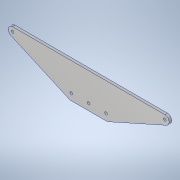
# Autodesk Inventor part: ハンド_上側板
Saved by Autodesk Inventor 2021 (Build 250183000, 183)
## iProperties
Created: 2021-12-06
Part Number: ハンド_上側板
Material: アルミニウム 6061
Document SubType Name: Modeling
Designer: 堀川皓史
Density: 2.7 g/cm^3
Appearance: アルミニウム - フラット
Mass: 47.8409 g
Surface Area: 131.403 cm^2
Volume: 17.7189 cm^3
Author: 堀川皓史
Autodesk Inventor part; units mm, degrees
ref_plane "YZ Plane" through (0, 0, 0) normal (1, 0, 0) x (0, 1, 0)
ref_plane "XZ Plane" through (0, 0, 0) normal (0, 1, 0) x (-1, 0, 0)
ref_plane "XY Plane" through (0, 0, 0) normal (0, 0, 1) x (1, 0, 0)
sketch "スケッチ1" plane through (0, 0, 0) normal (0, 0, 1) x (1, 0, 0)
  circle A0 centre (-20, 0) radius 1.6
  circle A1 centre (20, 0) radius 1.6
  circle A2 centre (0, 0) radius 1.6
  circle A3 centre (-87.5, 27.5) radius 1.6
  circle A4 centre (87.5, 27.5) radius 1.6
  arc A5 (-87.5, 32.5) -> (-89.5442, 22.937) centre (-87.5, 27.5) ccw
  arc A6 (89.5442, 22.937) -> (87.5, 32.5) centre (87.5, 27.5) ccw
  arc A7 (20, -7.5) -> (23.0663, -6.8445) centre (20, 0) ccw
  arc A8 (-23.0663, -6.8445) -> (-20, -7.5) centre (-20, 0) ccw
  line L0 (-89.5442, 22.937) -> (-23.0663, -6.8445)
  line L1 (-87.5, 32.5) -> (87.5, 32.5)
  line L2 (89.5442, 22.937) -> (23.0663, -6.8445)
  line L3 (20, -7.5) -> (-20, -7.5)
  dimension "d0" = 3.2
  dimension "d1" = 3.2
  dimension "d2" = 3.2
  dimension "d3" = 20
  dimension "d4" = 20
  dimension "d5" = 3.2
  dimension "d6" = 3.2
  dimension "d14" = 175
  dimension "d15" = 87.5
  dimension "d17" = 5
  dimension "d18" = 5
  dimension "d19" = 7.5
  dimension "d20" = 7.5
  dimension "d23" = 27.5
  constraints: 9 centre point, 8 end point, 8 point on circle, 8 tangent, 5 coincident, 3 horizontal alignment
  measures "d0" diameter of A0
  measures "d1" diameter of A1
  measures "d2" diameter of A2
  measures "d3" distance of point (0, 0) A0.centre
  measures "d4" distance of point (0, 0) A1.centre
  measures "d5" diameter of A3
  measures "d6" diameter of A4
  measures "d14" distance of A4.centre A3.centre
  measures "d15" horizontal distance of point (0, 0) A3.centre
  measures "d17" radius of A5
  measures "d18" radius of A6
  measures "d19" radius of A8
  measures "d20" radius of A7
  measures "d23" vertical distance of A0.centre A3.centre
extrude "押し出し1" add sketch "スケッチ1" along normal blind 3
equation "\"d15\" = 0.5 * d14"
